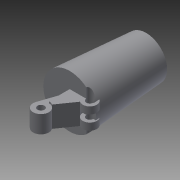
# Autodesk Inventor part: Ring_Upper_main_1
Saved by Autodesk Inventor 2015 (Build 190159000, 159)
## iProperties
Created: 2016-07-06
Part Number: Ring_Upper_main_1
Material: Generic
Document SubType Name: Modeling
Designer: Neelotpal Nag
Density: 1 g/cm^3
Appearance: Default
Author: Neelotpal Nag
Autodesk Inventor part; units mm, degrees
ref_plane "YZ Plane" through (0, 0, 0) normal (1, 0, 0) x (0, 1, 0)
ref_plane "XZ Plane" through (0, 0, 0) normal (0, 1, 0) x (-1, 0, 0)
ref_plane "XY Plane" through (0, 0, 0) normal (0, 0, 1) x (1, 0, 0)
sketch "Sketch1" plane through (0, 0, 0) normal (0, 0, 1) x (1, 0, 0)
  circle A0 centre (0, 0) radius 1
  circle A1 centre (0, 0) radius 2.25
  line L0 (0, 0) -> (2.25, 0) construction
  line L1 (0, 0) -> (0, 1)
  line L2 (0, 2.25) -> (0, 8.1915)
  circle A2 centre (5.7358, 8.1915) radius 1
  circle A3 centre (5.7358, 8.1915) radius 2
  line L3 (0, 0) -> (0.5736, 0.8192)
  line L4 (1.2905, 1.8431) -> (4.5886, 6.5532)
  line L5 (5.7358, 8.1915) -> (4.7358, 8.1915)
  line L6 (3.7358, 8.1915) -> (0, 8.1915)
  line L7 (9.3969, 13.4202) -> (9.3969, 8.1915)
  line L8 (9.3969, 8.1915) -> (7.7358, 8.1915)
  circle A4 centre (5.7358, 8.1915) radius 2.5
  line L9 (0, 0) -> (0, 30)
  line L10 (0, 30) -> (8.5505, 53.4923)
  line L11 (0, 30) -> (25, 30) construction
  circle A5 centre (0, 0) radius 2.5
  point P0 (17.9474, 50.0721)
  point P1 (8.5505, 53.4923)
  point P2 (17.9474, 50.0721)
  point P3 (-2.2437, 0.1688)
  dimension "d7" = 2
  dimension "d3" = 2
  dimension "d4" = 4.5
  dimension "d5" = 10
  dimension "d8" = 4
  dimension "d38" = 5
  dimension "d49" = 30
  dimension "d50" = 25
  dimension "d51" = 70
  dimension "d59" = 5
  constraints: 24 end point, 9 point on circle, 8 coincident, 5 centre point, 5 perpendicular, 4 vertical, 2 horizontal, 1 equal length, 1 horizontal alignment, 1 point on line, 2 other
  measures "d3" diameter of A0
  measures "d4" diameter of A1
  measures "d5" distance of L0.start L5.start
  measures "d8" diameter of A3
  measures "d38" diameter of A4
  measures "d49" distance of L0.start L9.end
  measures "d50" distance of L9.end L10.end
  measures "d51" angle of L11 L10
  measures "d59" diameter of A5
extrude "Extrusion1" add sketch "Sketch1" along normal mid plane 5 contours A3 | A2
extrude "Extrusion2" add sketch "Sketch1" along normal mid plane 6 contours A1 L2 A5 L4 | A5 L2 L6 A4 L4 | A4 L6 A3 L4 picked at (1.2382, 2.0622)
extrude "Extrusion4" add sketch "Sketch1" along normal mid plane 5 contours A1
sketch "Sketch2" plane through (0, 0, 2.5) normal (0, 0, 1) x (1, 0, 0)
  line L0 (0, 7.0508) -> (-2.1324, 0.718)
  arc A0 (0, 2.25) -> (1.2905, 1.8431) centre (0, 0) ccw projected
  line L1 (0, 7.0508) -> (0, 2.25)
  arc A1 (0, 2.25) -> (-2.1324, 0.718) centre (0, 0) ccw
  constraints: 4 end point, 3 point on circle, 1 centre point, 1 concentric, 1 tangent, 1 vertical
extrude "Extrusion5" add sketch "Sketch2" against normal blind 5
extrude "Extrusion6" add sketch "Sketch1" along normal mid plane 6 contours A3
extrude "Extrusion7" cut sketch "Sketch1" along normal mid plane 2 contours A3
sketch "Sketch3" plane through (0, 0, -1) normal (0, 0, 1) x (1, 0, 0)
  point P0 (0, 0)
extrude "Extrusion8" cut sketch "Sketch1" along normal mid plane 2 contours A4 L6 A3 L4 | L4 A3 L8 A4 | A4 L8 A3 L6
extrude "Extrusion11" add sketch "Sketch1" along normal mid plane 4 contours A1 L2 A5 L4 | A5 L2 L6 A4 L4 | A4 L6 A3 L4 picked at (1.2382, 2.0622)
sketch "Sketch6" plane through (0, 8.1915, -3) normal (0, 1, 0) x (1, 0, 0)
  circle A0 centre (0, -3) radius 7.5
  dimension "d52" = 15
  constraints: 1 centre point, 1 coincident
  measures "d52" diameter of A0
ref_plane "Work Plane1" through (0, 29.9915, -3) normal (0, 1, 0) x (1, 0, 0)
sketch "Sketch7" plane through (0, 29.9915, -3) normal (0, 1, 0) x (1, 0, 0)
  circle A0 centre (0, -3) radius 6
  dimension "d54" = 12
  constraints: 1 centre point, 1 coincident
  measures "d54" diameter of A0
loft "Loft1" add profiles "Sketch6", "Sketch7"
extrude "Extrusion13" cut sketch "Sketch1" along normal mid plane 20 contours A2
body "Solid1"
